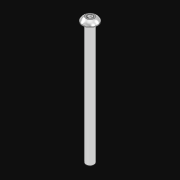
# Autodesk Inventor part: Screw 8-32 Steel 2.500
Saved by Autodesk Inventor 2021.3 (Build 253353010, 353A)
## iProperties
Created: 2020-07-03
Part Number: Screw 8-32 Steel 2.500
Material: VEX Steel
Document SubType Name: Modeling
Designer: yuany
Density: 1 g/cm^3
Appearance: Screws
Author: yuany
Autodesk Inventor part; units mm, degrees
ref_plane "YZ Plane" through (0, 0, 0) normal (1, 0, 0) x (0, 1, 0)
ref_plane "XZ Plane" through (0, 0, 0) normal (0, 1, 0) x (-1, 0, 0)
ref_plane "XY Plane" through (0, 0, 0) normal (0, 0, 1) x (1, 0, 0)
sketch "Sketch1" plane through (0, 0, 0) normal (0, 1, 0) x (-1, 0, 0)
  circle A0 centre (0, 0) radius 2.0828
  dimension "d4" = 4.1656
  constraints: 1 centre point, 1 coincident
  measures "d4" diameter of A0
extrude "Body" add sketch "Sketch1" along normal blind 63.5
sketch "Sketch2" plane through (0, 0, 0) normal (1, 0, 0) x (0, 1, 0)
  line L0 (63.5, -2.0828) -> (63.5, 2.0828) projected
  line L1 (63.5, 0) -> (63.5, -3.9624)
  line L2 (63.5, -3.9624) -> (63.881, -3.9624)
  arc A0 (63.881, -3.9624) -> (65.7098, -2.0828) centre (61.6888, 0) ccw
  line L3 (65.7098, -2.0828) -> (65.7098, -1.1938)
  line L4 (65.7098, -1.1938) -> (64.6176, -1.1938)
  line L5 (64.6176, -1.1938) -> (64.2366, -0.5588)
  line L6 (64.2366, -0.5588) -> (64.2366, 0)
  line L7 (64.2366, 0) -> (63.5, 0)
  point P0 (0, 0)
  dimension "d5" = 3.9624
  dimension "d6" = 0.381
  dimension "d13" = 0.7366
  dimension "d14" = 2.0828
  dimension "d15" = 2.2098
  dimension "d16" = 0
  dimension "d17" = 1.1938
  dimension "d18" = 0.5588
  dimension "d19" = 0.381
  constraints: 14 end point, 2 horizontal, 2 point on circle, 2 vertical, 1 centre point, 1 midpoint, 1 perpendicular, 1 point on line
  measures "d5" distance of L1.start L1.end
  measures "d6" distance of L1.end L2.end
  measures "d13" distance of L6.end L1.start
  measures "d14" distance from line of L3.start L7
  measures "d15" distance between parallel lines of L1 L3
  measures "d16" distance from line of L7 A0.centre
  measures "d17" distance from line of L3.end L7
  measures "d18" distance of L5.end L6.end
  measures "d19" distance from line of L4.end L6
revolve "Head" add sketch "Sketch2" angle 360 about axis through (0, 64.2366, 0) along (0, -1, 0)
sketch "Sketch3" plane through (0, 65.7098, 0) normal (0, 1, 0) x (1, 0, 0)
  line L0 (0.6892, 1.1938) -> (1.3785, 0)
  line L1 (1.3785, 0) -> (0.6892, -1.1938)
  line L2 (0.6892, -1.1938) -> (-0.6892, -1.1938)
  line L3 (-0.6892, -1.1938) -> (-1.3785, 0)
  line L4 (-1.3785, 0) -> (-0.6892, 1.1938)
  line L5 (-0.6892, 1.1938) -> (0.6892, 1.1938)
  circle A0 centre (0, 0) radius 1.1938 projected
  point P0 (0, 0)
  point P1 (0, 0)
  constraints: 12 end point, 1 coincident, 1 horizontal, 1 tangent, 13 other
extrude "Hex" cut sketch "Sketch3" against normal blind 1.1176
sketch "Sketch4" plane through (0, 0, 0) normal (0, 0, 1) x (1, 0, 0)
  line L0 (-0.6892, 64.5922) -> (0.6892, 64.5922) projected
  line L1 (-0.6892, 65.7098) -> (0.6892, 65.7098) projected
  line L2 (-0.254, 64.5922) -> (-1.3716, 65.7098)
  line L3 (-1.3785, 65.7098) -> (-1.3785, 64.5922) projected
  line L4 (-1.3785, 65.7098) -> (-0.254, 65.7098)
  line L5 (-0.254, 65.7098) -> (-0.254, 64.5922)
  line L6 (0, -6.792) -> (0, 40.7518) projected
  point P0 (0, 0)
  point P1 (0, 65.7098)
  dimension "d28" = 45
  dimension "d29" = 1.3716
  constraints: 6 end point, 2 point on line, 1 midpoint, 1 perpendicular
  measures "d28" angle of L0 L2
  measures "d29" distance of L2.end point (0, 65.71)
revolve "Head Chamfer" cut sketch "Sketch4" angle 360 about axis through (0, -10, 0) along (0, 1, 0)
sketch "Sketch5" plane through (0, 0, 0) normal (1, 0, 0) x (0, 1, 0)
  line L0 (0, -2.0828) -> (63.5, -2.0828) projected
  line L1 (63.5, 3.9624) -> (63.5, -3.9624) projected
  line L2 (63.5, -2.0828) -> (63.5, 2.0828) projected
  line L3 (0.0745, -2.0828) -> (-0.2261, -2.6035)
  line L4 (-0.2261, -2.6035) -> (-0.3253, -2.6035)
  line L5 (-0.3253, -2.6035) -> (-0.626, -2.0828)
  line L6 (0.0686, -2.6035) -> (-0.7252, -2.6035) construction
  line L7 (-0.626, -2.0828) -> (0.0745, -2.0828)
  line L8 (0, -2.0828) -> (63.5, -2.0828) projected
  point P0 (0, 0)
  dimension "d31" = 30
  dimension "d32" = 60
  dimension "a" = 0.0992
  dimension "d46" = 0.7937
  dimension "d54" = 0.0686
  dimension "d55" = 0.5207
  dimension "d56" = 0.0992
  constraints: 10 end point, 2 collinear, 2 point on line, 1 horizontal, 1 perpendicular
  measures "d31" angle of L1 L3
  measures "d32" angle of L3 L5
  measures "a" distance of L3.end L4.end
  measures "d46" distance of L6.start L6.end
  measures "d54" horizontal distance of L6.start L8.start
  measures "d55" distance between parallel lines of L4 L7
  measures "d56" horizontal distance of L5.end L6.end
feature "Thread" [suppressed]
sketch "Sketch6" plane through (0, 0, 0) normal (0, 0, 1) x (1, 0, 0)
  line L0 (0, 0) -> (-1.4859, 0)
  line L1 (2.0828, 0) -> (-2.0828, 0) projected
  line L2 (-1.4859, 0) -> (-2.4948, 1.0089)
  line L3 (-2.4948, 1.0089) -> (-2.9651, -1.2188)
  line L4 (-2.9651, -1.2188) -> (-1.4859, -1.2188)
  line L5 (-2.0828, 0) -> (-2.0828, 63.5) projected
  line L6 (-1.4859, -1.2188) -> (-1.4859, 0)
  line L7 (0, -7.8126) -> (0, 38.3438) projected
  point P0 (-2.0828, 0.5969)
  dimension "d49" = 1.4859
  dimension "d50" = 135
  constraints: 10 end point, 1 perpendicular, 1 point on line, 1 vertical
  measures "d49" distance from line of L0.start L6
  measures "d50" angle of L2 L6
revolve "Tapered End" cut sketch "Sketch6" angle 360 about axis through (0, -10, 0) along (0, 1, 0)
equation "\"d56\" = a"
body "Solid1"
